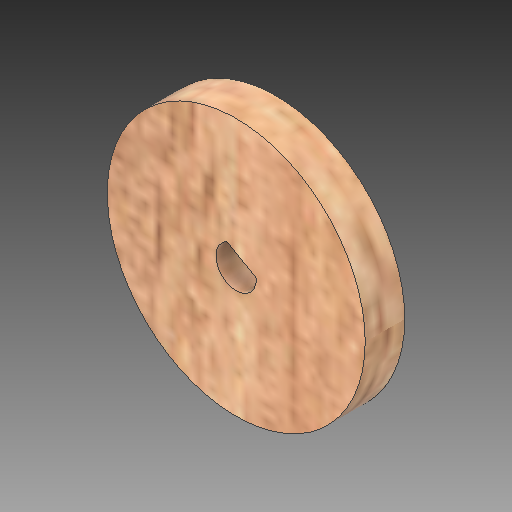
# Autodesk Inventor part: Knob
Saved by Autodesk Inventor 2018 (Build 220112000, 112)
## iProperties
Created: 2017-12-06
Part Number: Knob
Material: Wood (Birch)
Document SubType Name: Modeling
Designer: Andrew
Density: 0.55 g/cm^3
Appearance: Birch - Natural Polished
knobThick: 0.230 in
Author: Andrew
Autodesk Inventor part; units mm, degrees
ref_plane "YZ Plane" through (0, 0, 0) normal (1, 0, 0) x (0, 1, 0)
ref_plane "XZ Plane" through (0, 0, 0) normal (0, 1, 0) x (-1, 0, 0)
ref_plane "XY Plane" through (0, 0, 0) normal (0, 0, 1) x (1, 0, 0)
sketch "Sketch1" plane through (0, 0, 0) normal (0, 0, 1) x (1, 0, 0)
  circle A0 centre (0, 0) radius 19.05
  arc A1 (-1.3949, 2.6384) -> (2.9824, 0.1112) centre (0, 0) ccw
  line L0 (-1.3949, 2.6384) -> (2.9824, 0.1112)
  line L1 (-26.67, 0) -> (26.67, 0) projected
  dimension "d0" = 38.1
  dimension "d1" = 4.572
  dimension "d2" = 5.969
  dimension "d3" = 30
  constraints: 2 centre point, 2 coincident, 2 end point, 2 point on circle
  measures "d0" diameter of A0
  measures "d2" diameter of A1
  measures "d3" angle of L1 L0
derived "Enclosure Top.ipt"
extrude "Extrusion1" add sketch "Sketch1" along normal blind 5.842 contours L1 A1 L0 A0 | A0 L1 A1
equation "\"d5\" = knobThick"
equation "\"knobThick\" = 5.842"
body "Solid1"
